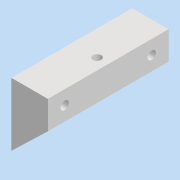
# Autodesk Inventor part: 23_Blocco_Escursione_Braccio_2
Saved by Autodesk Inventor 2020 (Build 240168000, 168)
## iProperties
Created: 2019-11-16
Part Number: 23_Blocco_Escursione_Braccio_2
Material: Generico
Document SubType Name: Modeling
Designer: socci
Density: 1 g/cm^3
Appearance: Default
Author: socci
Autodesk Inventor part; units mm, degrees
ref_plane "YZ Plane" through (0, 0, 0) normal (1, 0, 0) x (0, 1, 0)
ref_plane "XZ Plane" through (0, 0, 0) normal (0, 1, 0) x (-1, 0, 0)
ref_plane "XY Plane" through (0, 0, 0) normal (0, 0, 1) x (1, 0, 0)
sketch "Schizzo1" plane through (0, 0, 0) normal (0, 1, 0) x (-1, 0, 0)
  line L0 (30.1714, 73.6571) -> (4.1714, 73.6571)
  line L1 (4.1714, 73.6571) -> (4.1714, -12.3429)
  line L2 (4.1714, -12.3429) -> (30.1714, -12.3429)
  line L3 (30.1714, -12.3429) -> (30.1714, 73.6571)
  line L4 (30.1714, 73.6571) -> (4.1714, -12.3429) construction
  line L5 (4.1714, 73.6571) -> (30.1714, -12.3429) construction
  point P0 (0, 0)
  point P1 (17.1714, 30.6571)
  dimension "d0" = 26
  dimension "d1" = 86
  constraints: 12 end point, 2 midpoint, 2 parallel, 1 horizontal, 1 perpendicular
  measures "d0" distance of L1.end L2.end
  measures "d1" distance of L2.end L0.start
extrude "Estrusione1" add sketch "Schizzo1" along normal blind 20
sketch "Schizzo2" plane through (0, 0, 0) normal (0, -1, 0) x (1, 0, 0)
  line L0 (-4.1714, -12.3429) -> (-30.1714, -12.3429) projected
  line L1 (-4.1714, -12.3429) -> (-30.1714, -12.3429)
  line L2 (-30.1714, -12.3429) -> (-30.1714, 12.6571)
  line L3 (-30.1714, 12.6571) -> (-4.1714, 12.6571)
  line L4 (-4.1714, 12.6571) -> (-4.1714, -12.3429)
  line L5 (-30.1714, 73.6571) -> (-4.1714, 73.6571) projected
  line L6 (-4.1714, 73.6571) -> (-30.1714, 73.6571)
  line L7 (-30.1714, 73.6571) -> (-30.1714, 48.6571)
  line L8 (-30.1714, 48.6571) -> (-4.1714, 48.6571)
  line L9 (-4.1714, 48.6571) -> (-4.1714, 73.6571)
  point P0 (0, 0)
  dimension "d4" = 25
  dimension "d5" = 25
  constraints: 16 end point, 5 equal length, 2 perpendicular
  measures "d4" distance of L0.end L2.end
  measures "d5" distance of L7.end L5.start
extrude "Estrusione2" add sketch "Schizzo2" along normal blind 25
sketch "Schizzo3" plane through (-30.1714, 20, 73.6571) normal (0, 0, 1) x (1, 0, 0)
  line L0 (0, -20) -> (0, -45) projected
  line L1 (0, -45) -> (26, -45) projected
  line L2 (0, -45) -> (26, -45)
  line L3 (26, -20) -> (26, -45) projected
  line L4 (26, -45) -> (26, -20)
  line L5 (26, -20) -> (0, -45)
  point P0 (30.1714, -20)
  constraints: 6 end point, 2 collinear
extrude "Estrusione3" cut sketch "Schizzo3" against normal through all
sketch "Schizzo4" plane through (-4.1714, 20, 73.6571) normal (1, 0, 0) x (0, 0, -1)
  line L0 (86, 0) -> (0, 0) projected
  line L1 (0, 0) -> (0, -10)
  line L2 (0, -45) -> (0, 0) projected
  line L3 (0, 0) -> (10, 0) construction
  line L4 (0, -10) -> (12, -10)
  line L5 (86, 0) -> (86, -10)
  line L6 (86, -45) -> (86, 0) projected
  line L7 (86, 0) -> (96, 0) construction
  line L8 (86, -10) -> (74, -10)
  circle A0 centre (12, -10) radius 2.5
  circle A1 centre (74, -10) radius 2.5
  point P0 (73.6571, -20)
  dimension "d10" = 10
  dimension "d11" = 90
  dimension "d12" = 12
  dimension "d13" = 90
  dimension "d14" = 10
  dimension "d15" = 90
  dimension "d16" = 12
  dimension "d17" = 90
  dimension "d18" = 5
  dimension "d19" = 5
  constraints: 12 end point, 4 perpendicular, 2 centre point, 2 coincident, 2 collinear, 2 horizontal
  measures "d10" distance of L0.end L1.end
  measures "d11" angle of L1 L3
  measures "d12" distance of L1.end L4.end
  measures "d13" angle of L4 L1
  measures "d14" distance of L0.start L5.end
  measures "d15" angle of L5 L7
  measures "d16" distance of L5.end L8.end
  measures "d17" angle of L5 L8
  measures "d18" diameter of A0
  measures "d19" diameter of A1
hole "Foro1" at (-4.1714, 10, 61.6571) at (-4.1714, 10, -0.3429) direction (-1, 0, 0) diameter 5.9 end through all clearance for "Vite a testa piana" size "M5" standard "ANSI - Profilo M Metrico"
sketch "Schizzo5" plane through (0, 20, 0) normal (0, 1, 0) x (1, 0, 0)
  line L0 (-30.1714, -73.6571) -> (-4.1714, -73.6571) projected
  line L1 (-30.1714, 12.3429) -> (-30.1714, -73.6571) projected
  line L2 (-30.1714, -73.6571) -> (-30.1714, 12.3429)
  line L3 (-30.1714, -30.6571) -> (-12.1714, -30.6571)
  line L4 (-30.1714, -30.6571) -> (-12.1714, -30.6571) construction
  point P0 (0, 0)
  dimension "d27" = 18
  dimension "d28" = 0
  constraints: 6 end point, 2 coincident, 2 collinear, 2 horizontal, 1 midpoint
  measures "d27" distance of L3.start L3.end
  measures "d28" distance between parallel lines of L3 L4
hole "Foro2" at (-12.1714, 20, 30.6571) direction (0, -1, 0) diameter 5.9 end through all clearance for "Vite a testa piana" size "M5" standard "ANSI - Profilo M Metrico"
